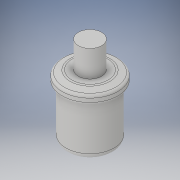
# Autodesk Inventor part: ConexionDireccionTop
Saved by Autodesk Inventor 2019 (Build 230136000, 136)
## iProperties
Created: 2019-12-22
Part Number: ConexionDireccionTop
Material: Generic
Document SubType Name: Modeling
Designer: Sergio
Density: 1 g/cm^3
Appearance: Default
Author: Sergio
Autodesk Inventor part; units mm, degrees
ref_plane "YZ Plane" through (0, 0, 0) normal (1, 0, 0) x (0, 1, 0)
ref_plane "XZ Plane" through (0, 0, 0) normal (0, 1, 0) x (-1, 0, 0)
ref_plane "XY Plane" through (0, 0, 0) normal (0, 0, 1) x (1, 0, 0)
sketch "Sketch1" plane through (0, 0, 0) normal (1, 0, 0) x (0, 1, 0)
  line L0 (31.0226, 0.1) -> (1.0226, 0.1)
  line L1 (1.0226, -8.025) -> (18.0226, -8.025)
  line L2 (18.0226, -8.025) -> (18.0226, -9.35)
  line L3 (18.0226, -9.35) -> (21.0226, -9.35)
  line L4 (22.0226, -3.85) -> (31.0226, -3.85)
  line L5 (31.0226, -3.85) -> (31.0226, 0.1)
  line L6 (1.0226, 0.1) -> (1.0226, -8.025)
  line L7 (51.327, 0.1) -> (-7.0634, 0.1) construction
  line L8 (22.0226, -3.85) -> (22.0226, -6.35)
  line L9 (22.0226, -6.35) -> (21.0226, -9.35)
  point P0 (0, 0)
  dimension "d0" = 3.95
  dimension "d2" = 3
  dimension "d4" = 9
  dimension "d5" = 30
  dimension "d7" = 8.125
  dimension "d11" = 2.5
  dimension "d12" = 1
  dimension "d14" = 0
  constraints: 20 end point, 2 horizontal, 2 perpendicular, 2 vertical, 1 parallel
  measures "d0" distance of L4.end L0.start
  measures "d2" distance of L2.end L3.end
  measures "d4" distance of L4.start L4.end
  measures "d5" distance of L0.start L0.end
  measures "d7" distance of L0.end L1.start
  measures "d11" distance of L4.start L8.end
  measures "d12" horizontal distance of L8.end L3.end
  measures "d14" distance between parallel lines of L7 L0
revolve "Revolution1" add sketch "Sketch1" angle 360 about axis through (0, 51.327, 0.1) along (0, -1, 0)
fillet "Fillet1" radius 1 2 edges at (0, 21.0226, 9.55) (0, 18.0226, 9.55)
fillet "Fillet3" radius 2 1 edges at (0, 1.0226, 8.225)
fillet "Fillet4" radius 2 1 edges at (0, 22.0226, 6.55)
body "Solid1"
